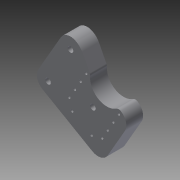
# Autodesk Inventor part: joint3+ax12imprint
Saved by Autodesk Inventor 2014 (Build 180170000, 170)
## iProperties
Created: 2014-01-12
Part Number: joint3+ax12imprint
Material: Générique
Document SubType Name: Modeling
Designer: helly
Density: 1 g/cm^3
Appearance: Par défaut
Author: helly
Autodesk Inventor part; units mm, degrees
ref_plane "YZ Plane" through (0, 0, 0) normal (1, 0, 0) x (0, 1, 0)
ref_plane "XZ Plane" through (0, 0, 0) normal (0, 1, 0) x (-1, 0, 0)
ref_plane "XY Plane" through (0, 0, 0) normal (0, 0, 1) x (1, 0, 0)
sketch "Esquisse1" plane through (0, 0, 0) normal (0, 1, 0) x (-1, 0, 0)
  line L0 (0, 0) -> (32, 0) construction
  line L1 (32, 0) -> (16, 27.7128) construction
  line L2 (16, 27.7128) -> (0, 0) construction
  line L3 (-10.3913, 17.9982) -> (9.0252, -15.6322) construction
  line L4 (8, -13.8564) -> (32, 0) construction
  line L5 (8, -13.8564) -> (14.9282, -9.8564) construction
  line L6 (8, -13.8564) -> (-10, 17.3205) construction
  line L7 (-10, 17.3205) -> (1.6913, 24.0705) construction
  line L8 (1.6913, 24.0705) -> (4.9413, 18.4413) construction
  line L9 (4.9413, 18.4413) -> (8.9413, 11.5131) construction
  line L10 (8.9413, 11.5131) -> (12.9413, 4.5849) construction
  line L11 (12.9413, 4.5849) -> (16.9413, -2.3433) construction
  circle A0 centre (8.9413, 11.5131) radius 1
  circle A1 centre (12.9413, 4.5849) radius 1
  circle A2 centre (16.9413, -2.3433) radius 1
  circle A3 centre (14.9282, -9.8564) radius 1
  circle A4 centre (4.9413, 18.4413) radius 1
  circle A5 centre (-14.4413, -1.9869) radius 1
  circle A6 centre (-10.4413, -8.9151) radius 1
  circle A7 centre (-6.4413, -15.8433) radius 1
  circle A8 centre (1.0718, -17.8564) radius 1
  circle A9 centre (-18.4413, 4.9413) radius 1
  circle A10 centre (-10, 17.3205) radius 11.6 construction
  line L12 (32, 0) -> (36, -6.9282) construction
  line L13 (36.0415, 0) -> (34.0207, -3.5) construction
  line L14 (34.0207, -3.5) -> (29.9793, -3.5) construction
  line L15 (29.9793, -3.5) -> (27.9585, 0) construction
  line L16 (27.9585, 0) -> (29.9793, 3.5) construction
  line L17 (29.9793, 3.5) -> (34.0207, 3.5) construction
  line L18 (34.0207, 3.5) -> (36.0415, 0) construction
  line L19 (34.0207, 3.5) -> (34.0207, -3.5) construction
  circle A11 centre (16, 27.7128) radius 2
  circle A12 centre (32, 0) radius 2
  line L20 (32, 0) -> (38.9282, 4) construction
  line L21 (-6.4413, -15.8433) -> (-13.3695, -19.8433) construction
  line L22 (42.9282, -2.9282) -> (-6.6195, -31.5346)
  line L23 (-6.6195, -31.5346) -> (-30.6195, 10.0346)
  line L24 (-30.6195, 10.0346) -> (18.9282, 38.641)
  line L25 (18.9282, 38.641) -> (42.9282, -2.9282)
  line L26 (8, -13.8564) -> (12, -20.7846) construction
  line L27 (16, 27.7128) -> (12, 34.641) construction
  circle A13 centre (0, 0) radius 2
  dimension "d0" = 32
  dimension "d1" = 32
  dimension "d2" = 60
  dimension "d4" = 8
  dimension "d6" = 36
  dimension "d7" = 13.5
  dimension "d8" = 6.5
  dimension "d9" = 8
  dimension "d10" = 8
  dimension "d11" = 8
  dimension "d13" = 2
  dimension "d14" = 11.6
  dimension "d15" = 8
  dimension "d16" = 7
  dimension "d17" = 4
  dimension "d19" = 8
  dimension "d20" = 8
  dimension "d26" = 8
  dimension "d27" = 8
  constraints: 56 end point, 14 centre point, 11 coincident, 11 point on line, 8 perpendicular, 6 equal radius, 5 collinear, 5 symmetric about line, 4 parallel, 1 horizontal, 18 other
  measures "d0" distance of L0.start L0.end
  measures "d1" distance of L0.end L1.end
  measures "d2" angle of L1 L0
  measures "d4" distance of L4.start L5.end
  measures "d6" distance of L4.start L6.end
  measures "d7" distance of L6.end L7.end
  measures "d8" distance of L7.end L8.end
  measures "d9" distance of L8.end L9.end
  measures "d10" distance of L9.end L10.end
  measures "d11" distance of L10.end L11.end
  measures "d13" diameter of A4
  measures "d14" radius of A10
  measures "d15" distance of L4.end L12.end
  measures "d16" distance of L17.end L13.end
  measures "d17" diameter of A11
  measures "d19" distance of L20.start L20.end
  measures "d20" distance of L21.start L21.end
  measures "d26" distance of L4.start L26.end
  measures "d27" distance of L27.start L27.end
extrude "Extrusion1" add sketch "Esquisse1" along normal blind 12
sketch "Esquisse5" plane through (0, 12, 0) normal (0, 1, 0) x (1, 0, 0)
  circle A0 centre (-32, 0) radius 2 projected
  circle A1 centre (-16, -27.7128) radius 2 projected
  line L0 (-42.9282, 2.9282) -> (-18.9282, -38.641) projected
  line L1 (-27.9585, 0) -> (-29.9793, -3.5)
  line L2 (-29.9793, -3.5) -> (-34.0207, -3.5)
  line L3 (-34.0207, -3.5) -> (-36.0415, 0)
  line L4 (-36.0415, 0) -> (-34.0207, 3.5)
  line L5 (-34.0207, 3.5) -> (-29.9793, 3.5)
  line L6 (-29.9793, 3.5) -> (-27.9585, 0)
  line L7 (-18.0207, -24.2128) -> (-13.9793, -24.2128)
  line L8 (-13.9793, -24.2128) -> (-11.9585, -27.7128)
  line L9 (-11.9585, -27.7128) -> (-13.9793, -31.2128)
  line L10 (-13.9793, -31.2128) -> (-18.0207, -31.2128)
  line L11 (-18.0207, -31.2128) -> (-20.0415, -27.7128)
  line L12 (-20.0415, -27.7128) -> (-18.0207, -24.2128)
  line L13 (-4.0415, 0) -> (-2.0207, 3.5)
  line L14 (-2.0207, 3.5) -> (2.0207, 3.5)
  line L15 (2.0207, 3.5) -> (4.0415, 0)
  line L16 (4.0415, 0) -> (2.0207, -3.5)
  line L17 (2.0207, -3.5) -> (-2.0207, -3.5)
  line L18 (-2.0207, -3.5) -> (-4.0415, 0)
  line L19 (-13.9793, -24.2128) -> (-20.0415, -27.7128) construction
  point P0 (0, 0)
  point P1 (0, 0)
  dimension "d51" = 7
  constraints: 38 end point, 3 coincident, 2 equal length, 2 parallel, 1 collinear, 39 other
  measures "d51" distance of L11.end L7.end
extrude "Extrusion2" cut sketch "Esquisse5" against normal blind 3
sketch "Esquisse6" plane through (0, 12, 0) normal (0, 1, 0) x (1, 0, 0)
  circle A0 centre (18.4413, -4.9413) radius 1 projected
  circle A1 centre (-4.9413, -18.4413) radius 1 projected
  line L0 (-18.9282, -38.641) -> (30.6195, -10.0346) projected
  line L1 (30.6195, -10.0346) -> (6.6195, 31.5346) projected
  line L2 (18.4413, -4.9413) -> (21.6913, -10.5705) construction
  line L3 (21.6913, -10.5705) -> (10, -17.3205) construction
  circle A2 centre (10, -17.3205) radius 12 construction
  line L4 (-11.9585, -27.7128) -> (-8.9689, -32.891) construction
  line L5 (-42.9282, 2.9282) -> (-18.9282, -38.641) projected
  circle A3 centre (-4.9413, -18.4413) radius 2.9833 construction
  line L6 (-8.9689, -32.891) -> (-2.2843, -19.7979)
  arc A4 (-2.2843, -19.7979) -> (-1.9664, -18.2182) centre (-4.9413, -18.4413) ccw
  circle A5 centre (18.4413, -4.9413) radius 2.9833 construction
  line L7 (19.933, -7.525) -> (26.8612, -3.525)
  arc A6 (16.7606, -7.4062) -> (-1.9664, -18.2182) centre (10, -17.3205) ccw
  arc A7 (16.7606, -7.4062) -> (19.933, -7.525) centre (18.4413, -4.9413) ccw
  point P0 (0, 0)
  dimension "d39" = 12
  dimension "d37" = 6.5
  dimension "d38" = 13.5
  constraints: 10 end point, 6 coincident, 6 point on circle, 3 centre point, 3 perpendicular, 3 point on line, 1 parallel, 11 other
  measures "d37" distance of L2.start L2.end
  measures "d38" distance of L2.end L3.end
extrude "Extrusion3" cut sketch "Esquisse6" against normal through all contours L6 A4 A6 A7 L7 L1 L0
fillet "Congé3" radius 10 1 edges at (-8.9689, 6, 32.891)
fillet "Congé4" radius 8 1 edges at (26.8612, 6, 3.525)
fillet "Congé5" radius 8 1 edges at (6.6195, 6, -31.5346)
fillet "Congé6" radius 8 1 edges at (-18.9282, 6, 38.641)
fillet "Congé7" radius 8 1 edges at (-42.9282, 6, -2.9282)
